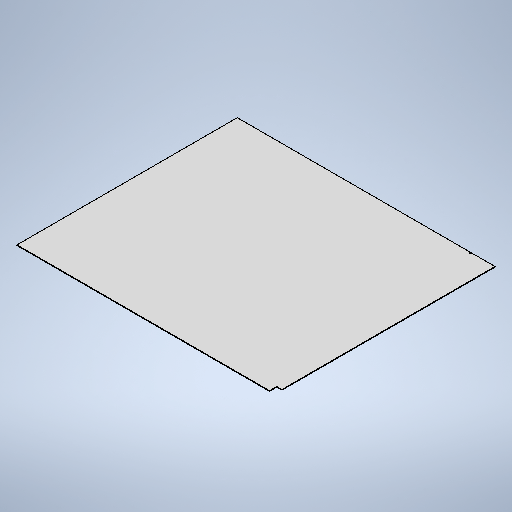
# Autodesk Inventor part: GnG frame 2 floor sheet 7
Saved by Autodesk Inventor 2025.3 (Build 293356000, 356)
## iProperties
Created: 2025-10-28
Part Number: GnG frame 2 floor sheet 7
Material: Stainless Steel
Document SubType Name: Sheet Metal
Designer: admin
Mass: 280.619 g
Surface Area: 364.406 cm^2
Volume: 35.0774 cm^3
Density: 8 g/cm^3
Sheet Metal Rule: AISI304 3mm Die 32
Sheet Metal Width: 1060,000 mm
Sheet Metal Length: 1240,000 mm
Sheet Metal Area: 1314400,000 mm^2
Appearance: Default
Flat Pattern Width: 106 cm
Flat Pattern Length: 124 cm
Flat Pattern Area: 13144 cm^2
Author: admin
Autodesk Inventor part; units mm, degrees
ref_plane "YZ Plane" through (0, 0, 0) normal (1, 0, 0) x (0, 1, 0)
ref_plane "XZ Plane" through (0, 0, 0) normal (0, 1, 0) x (-1, 0, 0)
ref_plane "XY Plane" through (0, 0, 0) normal (0, 0, 1) x (1, 0, 0)
sketch "Sketch1" plane through (0, 0, 0) normal (0, 0, 1) x (1, 0, 0)
  line L0 (0, 0) -> (-1240, 0)
  line L1 (-1240, 0) -> (-1240, -1060)
  line L2 (-1240, -1060) -> (0, -1060)
  line L3 (0, -1060) -> (0, 0)
  line L4 (0, 0) -> (-25, 0)
  line L5 (-25, 0) -> (-25, -35)
  line L6 (-25, -35) -> (0, -35)
  line L7 (0, -35) -> (0, 0)
  line L8 (0, -1060) -> (-25, -1060)
  line L9 (-25, -1060) -> (-25, -1025)
  line L10 (-25, -1025) -> (0, -1025)
  line L11 (0, -1025) -> (0, -1060)
  line L12 (-1240, 0) -> (-1215, 0)
  line L13 (-1215, 0) -> (-1215, -35)
  line L14 (-1215, -35) -> (-1240, -35)
  line L15 (-1240, -35) -> (-1240, 0)
  line L16 (-1240, -1060) -> (-1215, -1060)
  line L17 (-1215, -1060) -> (-1215, -1025)
  line L18 (-1215, -1025) -> (-1240, -1025)
  line L19 (-1240, -1025) -> (-1240, -1060)
  line L20 (-1085, -1060) -> (-995, -1060)
  line L21 (-995, -1060) -> (-995, -1025)
  line L22 (-995, -1025) -> (-1085, -1025)
  line L23 (-1085, -1025) -> (-1085, -1060)
  line L24 (-1085, 0) -> (-995, 0)
  line L25 (-995, 0) -> (-995, -35)
  line L26 (-995, -35) -> (-1085, -35)
  line L27 (-1085, -35) -> (-1085, 0)
  point P0 (0, -35)
  point P1 (-25, 0)
  point P2 (-25, -1060)
  point P3 (0, -1025)
  point P4 (-995, -1060)
  point P5 (-995, 0)
  dimension "d22" = 1240
  dimension "d23" = 1060
  dimension "d24" = 25
  dimension "d25" = 35
  dimension "d28" = 90
  dimension "d29" = 970
  measures "d22" distance of L2.end L1.end
  measures "d23" distance of L1.end L0.end
  measures "d24" distance of L6.end L5.end
  measures "d25" distance of L5.end L4.end
  measures "d28" distance of L25.end L26.end
  measures "d29" distance between parallel lines of L5 L25
extrude "Plate1" add sketch "Sketch1" along normal blind 3 contours L3 L6 L5 L0 | L5 L6 L3 L10 L9 L2 L21 L22 L23 L17 L18 L1 L14 L13 L0 L27 L26 L25 | L25 L26 L27 L0 | L13 L14 L1 L0 | L2 L23 L22 L21 | L18 L17 L2 L1
sketch "Sketch5" plane through (0, 0, 3) normal (0, 0, 1) x (1, 0, 0)
  line L0 (0, 0) -> (-100, 0) construction
  line L1 (-100, 0) -> (-100, -2) construction
  line L2 (-100, -2) -> (0, -2) construction
  line L3 (0, -2) -> (0, 0) construction
  line L4 (-100, 0) -> (-101.5248, -4.6556)
  arc A0 (-102.4752, -4.6556) -> (-101.5248, -4.6556) centre (-102, -4.5) ccw
  line L5 (-102.4752, -4.6556) -> (-104, 0)
  line L6 (-104, 0) -> (-100, 0)
  line L7 (-104, 0) -> (-106, 0) construction
  line L8 (-106, 0) -> (-108, 0)
  line L9 (-108, 0) -> (-108, -5)
  line L10 (-108, -5) -> (-106, -5)
  line L11 (-106, -5) -> (-106, 0)
  line L12 (-108, 0) -> (-110, 0) construction
  line L13 (-110, 0) -> (-112, 0)
  line L14 (-112, 0) -> (-112, -5)
  line L15 (-112, -5) -> (-110, -5)
  line L16 (-110, -5) -> (-110, 0)
  line L17 (-112, 0) -> (-114, 0) construction
  line L18 (-114, 0) -> (-116, 0)
  line L19 (-116, 0) -> (-116, -5)
  line L20 (-116, -5) -> (-114, -5)
  line L21 (-114, -5) -> (-114, 0)
  line L22 (-116, 0) -> (-118, 0) construction
  line L23 (-118, 0) -> (-120, 0)
  line L24 (-120, 0) -> (-120, -5)
  line L25 (-120, -5) -> (-118, -5)
  line L26 (-118, -5) -> (-118, 0)
  line L27 (-120, 0) -> (-125, 0) construction
  line L28 (-125, 0) -> (-130, 0) construction
  circle A1 centre (-125, 0) radius 1
  circle A2 centre (-130, 0) radius 1
  point P0 (-102, 0)
  dimension "d30" = 100
  dimension "d31" = 2
  dimension "d32" = 5
  dimension "d33" = 4
  dimension "d34" = 0.5
  dimension "d35" = 5
  dimension "d36" = 5
  dimension "d37" = 5
  dimension "d38" = 2
  constraints: 58 end point, 11 horizontal, 10 equal length, 10 parallel, 5 perpendicular, 4 coincident, 3 centre point, 3 tangent, 2 point on circle, 1 equal radius, 1 midpoint, 1 point on line, 1 vertical alignment
  measures "d30" distance of L2.end L1.end
  measures "d31" distance of L1.end L0.end
  measures "d32" distance of L9.end L9.start
  measures "d33" distance of L5.end L0.end
  measures "d34" radius of A0
  measures "d35" distance of L15.start L13.end
  measures "d36" distance of L19.end L19.start
  measures "d37" distance of L24.end L24.start
  measures "d38" diameter of A1
extrude "Cut1" cut sketch "Sketch5" against normal blind 3 contours L16 L15 L14 L13 | L21 L20 L19 L18 | L26 L25 L24 L23 | A1 | A2
equation "\"d33\" = 2 * d31"
equation "\"d34\" = 0.25 * d31"
equation "\"d38\" = d31"
equation "\"d39\" = Thickness"
equation "\"d2\" = Thickness"
equation "\"BendReliefWidth\" = Thickness"
equation "\"BendReliefDepth\" = 0.5 * Thickness"
equation "\"CornerReliefSize\" = 4 * Thickness"
equation "\"MinimumRemnant\" = 2 * Thickness"
equation "\"TransitionRadius\" = BendRadius"
equation "\"JacobiRadiusSize\" = BendRadius"
equation "\"GapSize\" = Thickness"
equation "\"Thickness\" = 3"
equation "\"BendRadius\" = 5"
body "Solid1"
